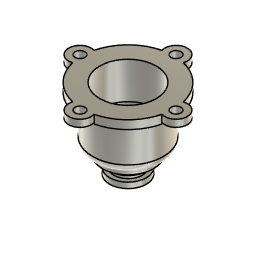
34 (Autodesk Fusion 360 design; units mm, degrees)
Autodesk Fusion 360 part; units mm, degrees
sketch "草图1" plane through (0, 0, 0) normal (0, 1, 0) x (1, 0, 0)
  line L0 (0, -75) -> (0, 50) construction
  line L1 (0, 56) -> (13, 56)
  line L2 (13, 56) -> (13, 52)
  line L3 (13, 52) -> (10, 52)
  line L4 (10, 52) -> (10, 48)
  line L5 (10, 48) -> (13, 48)
  line L6 (13, 48) -> (13, 44)
  line L7 (13, 44) -> (18, 44)
  line L8 (18, 44) -> (18, 40)
  arc A0 (25, 33) -> (18, 40) centre (18, 33) ccw
  line L9 (25, 33) -> (25, 6)
  line L10 (25, 6) -> (32.5, 6)
  line L11 (32.5, 6) -> (32.5, 0)
  line L12 (32.5, 0) -> (0, 0)
  line L13 (0, 56) -> (0, 0)
  line L14 (5, 56) -> (5, 36)
  line L15 (20, 26) -> (20, 0)
  line L16 (0, 0) -> (20, 0)
  line L17 (5, 36) -> (10, 36)
  arc A1 (20, 26) -> (10, 36) centre (10, 26) ccw
  dimension "d1" = 56
  dimension "d2" = 13
  dimension "d3" = 4
  dimension "d4" = 8
  dimension "d5" = 12
  dimension "d6" = 10
  dimension "d7" = 6
  dimension "d8" = 18
  dimension "d9" = 25
  dimension "d10" = 32.5
  dimension "d11" = 20
  dimension "d12" = 5
  dimension "d14" = 10
  dimension "d15" = 36
  dimension "d16" = 4
  constraint vertical L0
  constraint coincident L0 L1.start
  constraint perpendicular L0 L1
  constraint perpendicular L1 L2
  constraint perpendicular L2 L3
  constraint perpendicular L3 L4
  constraint perpendicular L4 L5
  constraint perpendicular L5 L6
  constraint perpendicular L6 L7
  constraint perpendicular L7 L8
  constraint perpendicular L9 L10
  constraint perpendicular L10 L11
  constraint coincident L0 L12.end
  constraint perpendicular L0 L12
  constraint tangent A0 L9
  constraint collinear L2 L6
  constraint coincident L12.end L13.end
  constraint coincident L1 L14.start
  constraint perpendicular L1 L14
  constraint coincident L12 L15.end
  constraint perpendicular L12 L15
  constraint perpendicular L0 L17
  constraint tangent L17 A1
  constraint tangent L15 A1
  constraint collinear L7.end L8.end A0.centre
  measures "d1" distance of L1.start L12.end
  measures "d2" distance of L1.start L1.end
  measures "d3" distance of L1.end L2.end
  measures "d4" vertical distance of L1.end L4.end
  measures "d5" vertical distance of L1.end L6.end
  measures "d6" horizontal distance of L1.start L3.end
  measures "d7" distance of L10.end L11.end
  measures "d8" horizontal distance of L1.start L7.end
  measures "d9" distance of L0 L9
  measures "d10" distance of L11.end L12.end
  measures "d11" distance of L12.end L15.end
  measures "d12" distance of L0 L14
  measures "d14" radius of A1
  measures "d15" distance of L16 L17
  measures "d16" distance of L7.end L8.end
revolve "旋转1" add sketch "草图1" angle 360 about axis through (0, 0, -56) along (0, 0, 1) contours L1 L2 L3 L4 L5 L6 L7 L8 A0 L9 L10 L11 L12 L14 L15 L17 A1 makes body 1
sketch "草图2" plane through (0, 0, -6) normal (0, 0, -1) x (1, 0, 0)
  circle A0 centre (0, 0) radius 25
  circle A1 centre (0, 0) radius 32.5
  circle A2 centre (0, 34) radius 8
  circle A3 centre (0, 34) radius 3.5
  line L0 (0, 50) -> (0, -40) construction
  circle A4 centre (-34, 0) radius 8
  circle A5 centre (-34, 0) radius 3.5
  circle A6 centre (0, -34) radius 8
  circle A7 centre (0, -34) radius 3.5
  circle A8 centre (34, 0) radius 8
  circle A9 centre (34, 0) radius 3.5
  dimension "d18" = 16
  dimension "d19" = 7
  dimension "d20" = 34
  dimension "d22" = 360
  constraint concentric A2 A3
  constraint vertical L0
  constraint collinear A0.centre A2.centre L0.start
  measures "d18" diameter of A2
  measures "d19" diameter of A3
  measures "d20" distance of A0.centre A2.centre
extrude "拉伸1" cut sketch "草图2" against normal blind 55 contours A1 A9 | A1 A8 A9 | A1 A8 A9 | A1 A2 A3 | A1 A2 A3 | A1 A6 A7 | A1 A6 A7 | A1 A3 | A1 A7 | A1 A4 A5 | A1 A5 picked at (31.855, 0.5938) picked at (0.084, 31.8255) picked at (-0.084, -31.8255) picked at (-30.8132, 4.3749) picked at (-31.8224, 0) bodies 1
extrude "拉伸2" add sketch "草图2" along normal blind 5 separate body contours A1 A8 A9 | A1 A8 A9 | A1 A2 A3 | A1 A2 A3 | A1 A6 A7 | A1 A6 A7 | A1 A4 A5 | A1 A4 A5 makes body 2 at (7.9602, -34.7965, -9.3333) makes body 3 at (-26.0398, 0.7965, -7.6667) makes body 4 at (41.9602, 0.7965, -7.6667) makes body 5 at (7.9602, 33.2035, -9.3333)
move_body "移动1" bodies 2 3 4 5 to x (1, 0, 0) y (0, 1, 0) z (0, 0, 1) at (0, 0, 6)
combine "合并1" operation add target body 5 tool bodies 1 3 2 4
